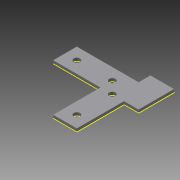
# Autodesk Inventor part: Gusset Connector
Saved by Autodesk Inventor 2013 (Build 170138000, 138)
## iProperties
Created: 2013-01-26
Part Number: Gusset Connector
Material: Generic
Document SubType Name: Modeling
Designer: actoennies
Density: 1 g/cm^3
Mass: 9.75912 g
Surface Area: 73.5882 cm^2
Volume: 9.75912 cm^3
Author: actoennies
Autodesk Inventor part; units mm, degrees
ref_plane "YZ Plane" through (0, 0, 0) normal (1, 0, 0) x (0, 1, 0)
ref_plane "XZ Plane" through (0, 0, 0) normal (0, 1, 0) x (-1, 0, 0)
ref_plane "XY Plane" through (0, 0, 0) normal (0, 0, 1) x (1, 0, 0)
sketch "Sketch1" plane through (0, 0, 0) normal (0, 1, 0) x (-1, 0, 0)
  line L0 (0, 0) -> (0, 76.2)
  line L1 (0, 76.2) -> (25.4, 76.2)
  line L2 (25.4, 76.2) -> (25.4, 25.4)
  line L3 (25.4, 25.4) -> (76.2, 25.4)
  line L4 (76.2, 25.4) -> (76.2, 0)
  line L5 (76.2, 0) -> (0, 0)
  line L6 (25.4, 25.4) -> (0, 0) construction
  circle A0 centre (12.7, 63.5) radius 3.3782
  circle A1 centre (12.7, 25.4) radius 3.3782
  circle A2 centre (25.4, 12.7) radius 3.3782
  circle A3 centre (63.5, 12.7) radius 3.3782
  dimension "d0" = 76.2
  dimension "d1" = 25.4
  dimension "d2" = 50.8
  dimension "d3" = 50.8
  dimension "d4" = 25.4
  dimension "d5" = 6.7564
  dimension "d6" = 6.7564
  dimension "d7" = 6.7564
  dimension "d8" = 6.7564
  dimension "d9" = 12.7
  dimension "d10" = 0
  dimension "d11" = 12.7
  dimension "d12" = 12.7
  dimension "d13" = 12.7
  dimension "d14" = 12.7
  dimension "d15" = 12.7
  constraints: 14 end point, 4 centre point, 4 point on line, 3 parallel, 1 perpendicular, 1 vertical
  measures "d0" distance of L0.end L6.end
  measures "d1" distance of L0.end L1.end
  measures "d2" distance of L1.end L2.end
  measures "d3" distance of L2.end L3.end
  measures "d4" distance of L3.end L4.end
  measures "d5" diameter of A0
  measures "d6" diameter of A1
  measures "d7" diameter of A2
  measures "d8" diameter of A3
  measures "d9" distance from line of L5 A2.centre
  measures "d10" distance from line of L3 A1.centre
  measures "d11" distance from line of L2 A1.centre
  measures "d12" distance from line of L4 A3.centre
  measures "d13" distance from line of L5 A3.centre
  measures "d14" distance from line of L1 A0.centre
  measures "d15" distance from line of L2 A0.centre
extrude "Extrusion1" add sketch "Sketch1" along normal blind 3.175
sketch "Sketch2" plane through (0, 0, 0) normal (0, -1, 0) x (1, 0, 0)
  line L0 (0, 76.2) -> (0, 0) projected
  line L1 (0, 0) -> (-76.2, 0) projected
  line L2 (0, 25.4) -> (15.621, 25.4)
  line L3 (15.621, 25.4) -> (15.621, -12.7)
  line L4 (15.621, -12.7) -> (-9.779, -12.7)
  line L5 (-9.779, -12.7) -> (-9.779, 0)
  dimension "d19" = 15.621
  dimension "d20" = 38.1
  dimension "d21" = 25.4
  constraints: 8 end point, 3 parallel, 2 point on line, 1 perpendicular
  measures "d19" distance of L2.start L2.end
  measures "d20" distance of L2.end L3.end
  measures "d21" distance of L3.end L4.end
extrude "Extrusion2" add sketch "Sketch2" against normal blind 3.175
sketch "Sketch3" plane through (0, 0, 0) normal (0, -1, 0) x (1, 0, 0)
  circle A0 centre (-63.5, 12.7) radius 3.3782 projected
  circle A1 centre (-25.4, 12.7) radius 3.3782 projected
  circle A2 centre (-12.7, 25.4) radius 3.3782 projected
  circle A3 centre (-12.7, 63.5) radius 3.3782 projected
  line L0 (0, 76.2) -> (0, 25.4) projected
  line L1 (-25.4, 76.2) -> (0, 76.2) projected
  line L2 (-25.4, 25.4) -> (-25.4, 76.2) projected
  line L3 (-76.2, 25.4) -> (-25.4, 25.4) projected
  line L4 (-76.2, 0) -> (-76.2, 25.4) projected
  line L5 (-9.779, 0) -> (-76.2, 0) projected
  line L6 (-9.779, 0) -> (-9.779, -12.7) projected
  line L7 (-9.779, -12.7) -> (15.621, -12.7) projected
  line L8 (15.621, -12.7) -> (15.621, 25.4) projected
  line L9 (15.621, 25.4) -> (0, 25.4) projected
  point P0 (0, 0)
body "Solid1"
